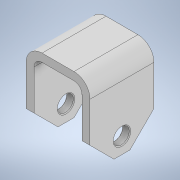
# Autodesk Inventor part: Blacha
Saved by Autodesk Inventor 2022 (Build 260153000, 153)
## iProperties
Created: 2024-01-14
Part Number: Blacha
Material: Generic
Document SubType Name: Modeling
Designer: mateu
Density: 1 g/cm^3
Appearance: Default
Author: mateu
Autodesk Inventor part; units mm, degrees
ref_plane "YZ Plane" through (0, 0, 0) normal (1, 0, 0) x (0, 1, 0)
ref_plane "XZ Plane" through (0, 0, 0) normal (0, 1, 0) x (-1, 0, 0)
ref_plane "XY Plane" through (0, 0, 0) normal (0, 0, 1) x (1, 0, 0)
sketch "Sketch1" plane through (0, 0, 0) normal (0, 0, 1) x (1, 0, 0)
  line L0 (0, 0) -> (0, 50)
  line L1 (0, 50) -> (-40, 50)
  line L2 (-40, 50) -> (-40, 0)
  line L3 (-40, 0) -> (-35, 0)
  line L4 (-35, 0) -> (-35, 45)
  line L5 (-35, 45) -> (-5, 45)
  line L6 (-5, 45) -> (-5, 0)
  line L7 (-5, 0) -> (0, 0)
  constraints: 16 end point, 4 perpendicular, 1 horizontal, 1 point on line, 1 vertical
extrude "Extrusion1" add sketch "Sketch1" along normal blind 40
fillet "Fillet1" radius 10 1 edges at (0, 50, 20)
fillet "Fillet2" radius 5 1 edges at (-5, 45, 20)
fillet "Fillet3" radius 10 1 edges at (-40, 50, 20)
fillet "Fillet4" radius 5 1 edges at (-35, 45, 20)
chamfer "Chamfer1" distance 15 angle 45 4 edges at (-2.5, 0, 40) (-2.5, 0, 0) (-37.5, 0, 40) (-37.5, 0, 0)
sketch "Sketch3" plane through (-40, 40, 0) normal (-1, 0, 0) x (0, 0, 1)
  point P0 (0, -40)
sketch "Sketch4" plane through (-40, 40, 0) normal (-1, 0, 0) x (0, 0, 1)
  line L0 (15, -40) -> (25, -40) projected
  point P0 (0, -40)
  point P1 (20, -30)
hole "Hole2" at (-40, 10, 20) direction (1, 0, 0) diameter 10 end through all
fillet "Fillet7" radius 0.5 4 edges at (-5, 10, 15) (-40, 10, 15) (0, 10, 15) (-35, 10, 15)
body "Solid1"
